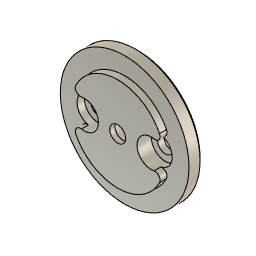
Apollo Yoke Disc P2 [(M)SPPS000000053] v1 (Autodesk Fusion 360 design; units mm, degrees)
Autodesk Fusion 360 part; units mm, degrees
sketch "Sketch1" plane through (0, 0, 0) normal (0, 1, 0) x (1, 0, 0)
  circle A0 centre (0, 0) radius 25
  circle A1 centre (-13, 0) radius 3
  circle A2 centre (13, 0) radius 3
  circle A3 centre (-13, 0) radius 5.5
  circle A4 centre (13, 0) radius 5.5
  circle A5 centre (0, 0) radius 18.25
  dimension "d1" = 50
  dimension "d2" = 26
  dimension "d3" = 13
  dimension "d4" = 6
  dimension "d5" = 6
  dimension "d17" = 11
  dimension "d18" = 11
  dimension "d41" = 36.5
  constraint coincident A0.centre A5.centre
  constraint horizontal A0.centre A1.centre
  constraint horizontal A0.centre A2.centre
  constraint concentric A1 A3
  constraint concentric A2 A4
  measures "d1" diameter of A0
  measures "d2" distance of A1.centre A2.centre
  measures "d3" distance of A0.centre A2.centre
  measures "d4" diameter of A1
  measures "d5" diameter of A2
  measures "d17" diameter of A3
  measures "d18" diameter of A4
  measures "d41" diameter of A5
extrude "Extrude1" add sketch "Sketch1" along normal blind 8 contours A0 | A3 A5 | A3 A4 A5 | A3 A5 | A4 A5 | A4 A5
sketch "Sketch2" plane through (0, 8, 0) normal (0, 1, 0) x (-1, 0, 0)
  circle A0 centre (13, 0) radius 3
  circle A1 centre (-13, 0) radius 3
  circle A2 centre (0, 0) radius 3
  circle A3 centre (0, 0) radius 25
  circle A4 centre (0, 0) radius 6.3
  dimension "d26" = 6
  dimension "d37" = 12.6
  constraint coincident A2.centre A3.centre
  constraint concentric A3 A4
  measures "d26" diameter of A2
  measures "d37" diameter of A4
hole "Hole1" at (0, 8, 0) direction (0, -1, 0) diameter 6.2 depth 9 tip angle 118 counterbore diameter 12.4 counterbore depth 6
extrude "Extrude2" cut sketch "Sketch1" along normal blind 5.5 contours A3 A5 | A3 A5 | A4 A5 | A4 A5
extrude "Extrude4" cut sketch "Sketch1" along normal blind 2.7 contours A0
chamfer "Chamfer1" distance 1 angle 45 1 edges at (-23.3082, 8, 9.0404)
fillet "Fillet1" radius 2 4 edges at (-18.1466, 1.35, 1.9396) (-18.1466, 1.35, -1.9396) (18.1466, 1.35, 1.9396) (18.1466, 1.35, -1.9396)
sketch "Sketch3" plane through (0, 0, 0) normal (0, -1, 0) x (1, 0, 0)
  arc A0 (16.2765, -8.2545) -> (14.0947, -5.39) centre (14.4928, -7.3499) ccw
  arc A1 (14.0947, 5.39) -> (14.0947, -5.39) centre (13, 0) ccw
  arc A2 (14.0947, 5.39) -> (16.2765, 8.2545) centre (14.4928, 7.3499) ccw
  arc A3 (16.2765, 8.2545) -> (-16.2765, 8.2545) centre (0, 0) ccw
  arc A4 (-16.2765, 8.2545) -> (-14.0947, 5.39) centre (-14.4928, 7.3499) ccw
  arc A5 (-14.0947, -5.39) -> (-14.0947, 5.39) centre (-13, 0) ccw
  arc A6 (-14.0947, -5.39) -> (-16.2765, -8.2545) centre (-14.4928, -7.3499) ccw
  arc A7 (-16.2765, -8.2545) -> (16.2765, -8.2545) centre (0, 0) ccw
  circle A8 centre (0, 0) radius 3.1
  circle A9 centre (0, 0) radius 18.25
  dimension "d46" = 36.5
  constraint coincident A3.centre A7.centre
  measures "d46" diameter of A9
sketch "Sketch4" plane through (0, 0, 0) normal (0, -1, 0) x (1, 0, 0)
  arc A0 (16.2765, -8.2545) -> (14.0947, -5.39) centre (14.4928, -7.3499) ccw
  arc A1 (14.0947, 5.39) -> (14.0947, -5.39) centre (13, 0) ccw
  arc A2 (14.0947, 5.39) -> (16.2765, 8.2545) centre (14.4928, 7.3499) ccw
  arc A3 (16.2765, 8.2545) -> (-16.2765, 8.2545) centre (0, 0) ccw
  arc A4 (-16.2765, 8.2545) -> (-14.0947, 5.39) centre (-14.4928, 7.3499) ccw
  arc A5 (-14.0947, -5.39) -> (-14.0947, 5.39) centre (-13, 0) ccw
  arc A6 (-14.0947, -5.39) -> (-16.2765, -8.2545) centre (-14.4928, -7.3499) ccw
  arc A7 (-16.2765, -8.2545) -> (16.2765, -8.2545) centre (0, 0) ccw
  circle A8 centre (0, 0) radius 3.1
  line L0 (30, 27.5) -> (-30, 27.5)
  line L1 (-30, 27.5) -> (-30, -27.5)
  line L2 (-30, -27.5) -> (30, -27.5)
  line L3 (30, -27.5) -> (30, 27.5)
  line L4 (30, 27.5) -> (-30, -27.5) construction
  line L5 (-30, 27.5) -> (30, -27.5) construction
  dimension "d47" = 60
  dimension "d48" = 55
  constraint horizontal L0
  constraint perpendicular L0 L1
  constraint parallel L0 L2
  constraint parallel L1 L3
  constraint coincident L4 A3.centre
  constraint coincident L5 A3.centre
  constraint coincident A3.centre A7.centre
  measures "d47" distance of L1.end L2.end
  measures "d48" distance of L0.end L1.end
equation "d3 = d2 / 2"
